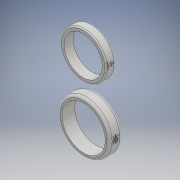
# Autodesk Inventor part: Rings
Saved by Autodesk Inventor 2018 (Build 220112000, 112)
## iProperties
Created: 2021-07-04
Part Number: Rings
Material: Generic
Document SubType Name: Modeling
Designer: dangl
Density: 1 g/cm^3
Appearance: Default
Author: dangl
Autodesk Inventor part; units mm, degrees
ref_plane "XZ Plane" through (0, 0, 0) normal (0, 1, 0) x (-1, 0, 0)
ref_plane "XY Plane" through (0, 0, 0) normal (0, 0, 1) x (1, 0, 0)
sketch "Sketch1" plane through (0, 0, 0) normal (0, 1, 0) x (-1, 0, 0)
  circle A0 centre (0, 0) radius 8.5
  circle A1 centre (0.2028, 24.5776) radius 7.5
  circle A2 centre (0.2028, 24.5776) radius 9
  circle A3 centre (0, 0) radius 10.2
  dimension "d0" = 17
  dimension "d1" = 15
  dimension "d2" = 1.5
  dimension "d3" = 1.7
  constraints: 4 centre point, 1 coincident
  measures "d0" diameter of A0
  measures "d1" diameter of A1
  measures "d2" radial gap between concentric circles of A1 A2
  measures "d3" radial gap between concentric circles of A0 A3
extrude "Extrusion1" add sketch "Sketch1" along normal blind 5 contours A3
extrude "Extrusion2" add sketch "Sketch1" along normal blind 3.6 contours A2
fillet "Fillet1" radius 0.5 2 edges at (8.7972, 3.6, 24.5776) (8.7972, 0, 24.5776)
fillet "Fillet2" radius 1 2 edges at (10.2, 0, 0) (10.2, 5, 0)
ref_plane "Work Plane1" through (14.75, 0, 0) normal (1, 0, 0) x (0, 1, 0)
sketch "Sketch2" plane through (14.75, 0, 0) normal (1, 0, 0) x (0, 1, 0)
  line L0 (2.9528, 26.9029) -> (2.9528, 22.7113) construction
  line L1 (2.9528, 22.7113) -> (-0.5176, 22.7113) construction
  line L2 (-0.5176, 22.7113) -> (-0.5176, 26.9029) construction
  line L3 (-0.5176, 26.9029) -> (2.9528, 26.9029) construction
  line L4 (3.8215, 1.853) -> (3.8215, -2.3386) construction
  line L5 (3.8215, -2.3386) -> (0.3512, -2.3386) construction
  line L6 (0.3512, -2.3386) -> (0.3512, 1.853) construction
  line L7 (0.3512, 1.853) -> (3.8215, 1.853) construction
  spline S0 degree 2 poles (0.9157, 25.0073) (0.9673, 24.5014) (1.0339, 24.0204) (0.9207, 23.7075) (0.6927, 23.6626) (0.7576, 24.2351) (0.706, 25.2303) (0.5762, 26.0425) (0.5096, 26.3421) (0.8125, 26.7065) (0.7975, 26.2322) (0.8508, 25.6231) (0.9124, 25.1704) knots 0 0 0 1 2 3 4 5 6 7 8 9 10 11 11 11
  spline S1 degree 2 poles (0.9124, 25.1704) (1.3418, 24.994) (1.7079, 24.8659) (1.9609, 24.8925) (1.8643, 24.6312) (1.6896, 24.4465) (1.5381, 24.6495) (0.9157, 25.0073) knots 0 0 0 1 2 3 4 5 6 6 6
  spline S2 degree 2 poles (2.1905, 25.2603) (2.2737, 24.8892) (2.3653, 24.5314) (2.2538, 24.2368) (2.104, 24.3732) (2.0241, 24.9108) (1.9226, 25.4067) (1.8677, 25.6997) (2.0657, 26.0541) (2.1156, 25.5848) (2.1905, 25.2603) knots 0 0 0 1 2 3 4 5 6 7 8 9 9 9
  spline S3 degree 2 poles (2.8712, 25.0007) (2.7963, 24.8243) (2.4551, 24.8559) (2.59, 25.1771) (2.7381, 25.3785) (2.9528, 25.5199) (2.9528, 25.3285) knots 0 0 0 1 2 3 4 5 5 5
  spline S4 degree 2 poles (2.9528, 25.3285) (2.9528, 25.1505) (2.8712, 25.0007) knots 0 0 0 1 1 1
  spline S5 degree 2 poles (1.4732, 25.7463) (1.7512, 25.8578) (1.5465, 25.4467) (1.3418, 25.3335) (1.0455, 25.465) (1.2719, 25.6464) (1.4732, 25.7463) knots 0 0 0 1 2 3 4 5 5 5
  spline S6 degree 2 poles (2.362, -0.68) (2.1373, -0.6683) (1.633, -0.5618) (1.3085, -0.3455) (1.1571, -0.0276) (1.5315, -0.2905) (2.0957, -0.4703) (2.3437, -0.4836) knots 0 0 0 1 2 3 4 5 6 6 6
  spline S7 degree 2 poles (2.3437, -0.4836) (2.3204, -0.3338) (2.3087, -0.2523) knots 0 0 0 1 1 1
  spline S8 degree 2 poles (2.3087, -0.2523) (1.9809, -0.2523) (1.5465, -0.2639) (1.3002, -0.0958) (1.5332, 0.0323) (1.7445, 0.247) (1.7063, 0.054) (1.7162, -0.0426) (1.9376, -0.0659) (2.2921, -0.0659) knots 0 0 0 1 2 3 4 5 6 7 8 8 8
  spline S9 degree 2 poles (2.2921, -0.0659) (2.2788, 0.0007) (2.2588, 0.1022) knots 0 0 0 1 1 1
  spline S10 degree 2 poles (2.2588, 0.1022) (1.886, 0.1139) (1.4267, 0.3569) (1.2602, 0.6914) (1.445, 0.5666) (1.6613, 0.4268) (1.9925, 0.3119) (2.2272, 0.287) knots 0 0 0 1 2 3 4 5 6 6 6
  spline S11 degree 2 poles (2.2272, 0.287) (2.2155, 0.3319) (2.2005, 0.46) (2.3853, 0.6131) (2.3853, 0.4883) knots 0 0 0 1 2 3 3 3
  spline S12 degree 2 poles (2.3853, 0.4883) (2.3853, 0.3968) (2.4052, 0.2853) knots 0 0 0 1 1 1
  spline S13 degree 2 poles (2.4052, 0.2853) (2.5866, 0.2736) (3.0709, 0.287) (3.2457, 0.3901) (3.2324, 0.1804) (3.2207, 0.1472) (3.244, 0.0074) (3.3256, -0.0942) (3.254, -0.2622) (3.1658, -0.3554) (3.0443, -0.2772) (2.7098, -0.2523) (2.4768, -0.2523) knots 0 0 0 1 2 3 4 5 6 7 8 9 10 11 11 11
  spline S14 degree 2 poles (2.4768, -0.2523) (2.4885, -0.3388) (2.5101, -0.4836) knots 0 0 0 1 1 1
  spline S15 degree 2 poles (2.5101, -0.4836) (2.7414, -0.4836) (3.1242, -0.4703) (3.3256, -0.3654) (3.3106, -0.5635) (3.2856, -0.6367) (3.3222, -0.8031) (3.3905, -0.903) (3.3339, -1.0827) (3.2207, -1.2175) (3.0843, -1.1376) (2.8679, -1.126) (2.6199, -1.126) knots 0 0 0 1 2 3 4 5 6 7 8 9 10 11 11 11
  spline S16 degree 2 poles (2.6199, -1.126) (2.6466, -1.2209) (2.6316, -1.3573) (2.4402, -1.4921) (2.4236, -1.2541) (2.4119, -1.126) knots 0 0 0 1 2 3 4 4 4
  spline S17 degree 2 poles (2.4119, -1.126) (2.0707, -1.126) (1.4866, -1.1659) (1.2153, -1.1243) (1.0123, -0.923) (1.2885, -0.8148) (1.5631, -0.5884) (1.5082, -0.7898) (1.4716, -0.893) (1.6763, -0.9146) (1.856, -0.9146) knots 0 0 0 1 2 3 4 5 6 7 8 9 9 9
  line L8 (1.856, -0.9146) -> (2.3969, -0.9146)
  spline S18 degree 2 poles (2.3969, -0.9146) (2.3853, -0.8564) (2.362, -0.68) knots 0 0 0 1 1 1
  spline S19 degree 2 poles (2.6798, 0.708) (2.7198, 0.6914) (2.9728, 0.743) (2.7947, 0.3885) (2.6399, 0.4684) (2.4202, 0.5466) (2.094, 0.6115) (1.8893, 0.7147) knots 0 0 0 1 2 3 4 5 6 6 6
  spline S20 degree 2 poles (1.8893, 0.7147) (1.7828, 0.5898) (1.6197, 0.5183) (1.3917, 0.6414) (1.6647, 0.8162) (1.7046, 0.8395) knots 0 0 0 1 2 3 4 4 4
  spline S21 degree 2 poles (1.7046, 0.8395) (1.5964, 0.921) (1.3817, 1.2023) (1.2602, 1.605) (1.5032, 1.3304) (1.7329, 1.0492) (1.866, 0.966) knots 0 0 0 1 2 3 4 5 5 5
  spline S22 degree 2 poles (1.866, 0.966) (2.0374, 1.1108) (2.114, 1.2139) (2.2122, 1.2006) (2.3969, 1.1474) knots 0 0 0 1 2 3 3 3
  spline S23 degree 2 poles (2.3969, 1.1474) (2.3204, 1.3504) (2.2272, 1.5535) (2.5151, 1.7881) (2.4901, 1.5102) (2.5883, 1.1174) knots 0 0 0 1 2 3 4 4 4
  spline S24 degree 2 poles (2.5883, 1.1174) (2.9844, 1.0309) (3.4604, 0.9776) (3.5869, 0.9909) (3.8215, 1.0442) (3.7383, 0.7979) (3.6434, 0.6614) (3.4254, 0.7413) (2.6199, 0.9227) knots 0 0 0 1 2 3 4 5 6 7 7 7
  line L9 (2.6199, 0.9227) -> (2.6798, 0.708)
  spline S25 degree 2 poles (2.5284, -0.6816) (2.5517, -0.7765) (2.5866, -0.9146) knots 0 0 0 1 1 1
  spline S26 degree 2 poles (2.5866, -0.9146) (3.051, -0.9146) (3.1791, -0.883) (3.1675, -0.8497) knots 0 0 0 1 2 2 2
  line L10 (3.1675, -0.8497) -> (3.1342, -0.6816)
  line L11 (3.1342, -0.6816) -> (2.5284, -0.6816)
  spline S27 degree 2 poles (2.4369, 0.1006) (2.4485, 0.0007) (2.4585, -0.0659) knots 0 0 0 1 1 1
  line L12 (2.4585, -0.0659) -> (3.056, -0.0659)
  spline S28 degree 2 poles (3.056, -0.0659) (3.1009, -0.0659) (3.1009, -0.0476) knots 0 0 0 1 1 1
  spline S29 degree 2 poles (3.1009, -0.0476) (3.1009, 0.0007) (3.0809, 0.1006) knots 0 0 0 1 1 1
  line L13 (3.0809, 0.1006) -> (2.4369, 0.1006)
  spline S30 degree 2 poles (2.4452, 0.941) (2.2405, 0.9893) (2.1423, 1.0009) (2.089, 0.9477) (2.0191, 0.8778) knots 0 0 0 1 2 3 3 3
  spline S31 degree 2 poles (2.0191, 0.8778) (2.1922, 0.7946) (2.54, 0.7296) knots 0 0 0 1 1 1
  spline S32 degree 2 poles (2.54, 0.7296) (2.5034, 0.7896) (2.4452, 0.941) knots 0 0 0 1 1 1
  point P0 (0, 0)
  constraints: 4 other
emboss "Emboss1" sketch "Sketch2" operation cut depth 1 direction (-1, 0, 0) contours S0 S1 | S2 | S3 S4 | S5
emboss "Emboss2" sketch "Sketch2" operation cut depth 1 direction (-1, 0, 0) contours S6 S7 S8 S9 S10 S11 S19 S12 S13 S14 S15 S16 S17 L8 S18 | S19 S20 S21 S22 S23 S24 L9 S11 | S11 S19
body "Solid1"
